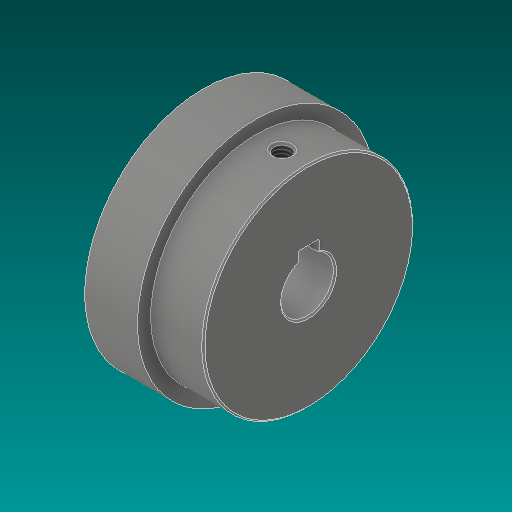
# Autodesk Inventor part: GEYK1.0-70-10-B-10K.0_b
Saved by Autodesk Inventor 2020 (Build 240168000, 168)
## iProperties
Created: 2022-11-14
Part Number: GEYK1.0-70-10-B-10K.0_b
Material: Generic
Catalog Web Link: www.cadenas.de
Description: GEY_body-Plastic Bonded Spur Gears
Vendor: MISUMI
Document SubType Name: Modeling
Designer: psAdmin
Manufacturer: MISUMI
Mass: 26.6277 g
Surface Area: 64.7379 cm^2
Volume: 26.6277 cm^3
Density: 1 g/cm^3
Appearance: PSOLRGB-128-128-128
Category: PARTsolutions
Company: MISUMI
PSOL_IDENT_0: {$CADENAS_DATA/23d-libs/misumi/metric/54_spur_gears/gey_.prj},213 {VTYP=3D},{NB=GEYK1.0-70-10-B-10K.
PSOL_IDENT_1: 0_b},{LINA=GEYK1.0-70-10-B-10K.0},{NN=GEY_body},{DATE=07.06.2021 01:25:59},{GEOMDATE=23.08.2016 05:0
PSOL_IDENT_2: 9:00},{VERSION=},{LINEID=10},{WBVAR=SHS,NT,PS,ALT1,ALT2,BS},{WBNUMERIC=NT,BS}  {NB=GEYK1.0-70-10-B-1
PSOL_IDENT_3: 0K.0_b},{LINA=GEYK1.0-70-10-B-10K.0},{KT=DUMMY},{PN=GEYK1.0-70-10-B-10K.0},{SHS=K},{SHSPN=K},{GEAKBH=
PSOL_IDENT_4: 0},{MAT=MC Nylon},{MATC=S25C},{AC=Set Screw},{MOD=1.0},{NT=70},{NTA=30,32,34,35,36,38,40,42,45,48,50
PSOL_IDENT_5: ,52,56,60,70,75},{B=10},{TS=B},{TSA='B','B'},{PS=10K},{PSA= '10N','10N','10K','10K','11N','11N','12N'
PSOL_IDENT_6: ,'12N','13N','13N','14N','14N','15N','15N','16N','16N','17N','17N','18N','18N','19N','19N','20N','20
PSOL_IDENT_7: N','21N','21N','22N','22N','23N','23N','24N','24N'},{PS1= '10','10','11','11','12','12','13','13','1
PSOL_IDENT_8: 4','14','15','15','16','16','17','17','18','18','19','19','20','20','21','21','22','22','23','23','2
PSOL_IDENT_9: 4','24','25','25','26','26','27','27','28','28'},{PS2= '10N','10N','10K','10K','11N','11N','12N','12
PSOL_IDENT_10: N','13N','13N','14N','14N','15N','15N','16N','16N','17N','17N','18N','18N','19N','19N','20N','20N','
PSOL_IDENT_11: 21N','21N','22N','22N','23N','23N','24N','24N'},{P=10.00},{DD=70.0},{D=72.0},{H=40},{E=45},{L=20},{L
PSOL_IDENT_12: L1=10},{LL2=5.000},{M=M4},{M2=4},{ACSS=M4x3},{TT=1.8},{BB=4},{ALT1=},{ALTA='','w/o Set Screw', '-KC9
PSOL_IDENT_13: 0', 'with KC90 (Set Screw)', '-KC120', 'with KC120 (Set Screw)'},{SCREWL=3},{PLANE=20},{PLANE1=20},{
PSOL_IDENT_14: ALT2=},{ALT2A='','w/o Boss Cut','-BS','with BS (Boss Cut)'},{BS=0.0},{BSA=0},{BSMIN=7.0},{BSMAX=9.5}
PSOL_IDENT_15: ,{HD=15.000}
NB: GEYK1.0-70-10-B-10K.0_b
NN: GEY_body
NT: 70
NBSYN: $PN._b
LINA: GEYK1.0-70-10-B-10K.0
CATALOG: Misumi
PN: GEYK1.0-70-10-B-10K.0
SHS: Key Groove Hole+Tap
MAT: MC Nylon
MATC: S25C
MOD: 1.0
B: 10
PS: 10K
L: 20
LL1: 10
ALT1: w/o Set Screw
ALT2: w/o Boss Cut
BS: 0
SUPPLIER: MISUMI
ARTICLENO: GEYK1.0-70-10-B-10K.0_b
BOMINFO: GEYK1.0-70-10-B-10K.0
CREATOR: CADENAS GmbH
d9: 0.000 mm
Title: GEYK1.0-70-10-B-10K.0
Author: Cadenas PARTsolutions
Comments: Plastic Bonded Spur Gears
Autodesk Inventor part; units mm, degrees
ref_plane "YZ Plane" through (0, 0, 0) normal (1, 0, 0) x (0, 1, 0)
ref_plane "XZ Plane" through (0, 0, 0) normal (0, 1, 0) x (-1, 0, 0)
ref_plane "XY Plane" through (0, 0, 0) normal (0, 0, 1) x (1, 0, 0)
sketch "Sketch_11" plane through (0, 0, 0) normal (0, 0, 1) x (1, 0, 0)
  line L0 (20, 0) -> (0, 0)
  line L1 (0, 0) -> (0, 34)
  line L2 (0, 34) -> (0.5359, 36)
  line L3 (0.5359, 36) -> (9.4641, 36)
  line L4 (9.4641, 36) -> (10, 34)
  line L5 (10, 34) -> (10, 20)
  line L6 (10, 20) -> (19.7, 20)
  line L7 (19.7, 20) -> (20, 19.7)
  line L8 (20, 19.7) -> (20, 0)
  line L9 (20, 0) -> (0, 0)
  constraints: 20 end point
revolve "Revolution1" add sketch "Sketch_11" angle 360 about axis through (20, 0, 0) along (1, 0, 0)
sketch "Sketch_2" plane through (0, 0, 0) normal (1, 0, 0) x (0, 1, 0)
  circle A0 centre (0, 0) radius 41
  circle A1 centre (0, 0) radius 22.5
  constraints: 2 centre point
extrude "Extrusion1" cut sketch "Sketch_2" along normal blind 10
sketch "_____1" plane through (0, 0, 0) normal (0, 0, 1) x (1, 0, 0)
  line L0 (40, 0) -> (-40, 0)
  line L1 (0, 0) -> (0, 5.3)
  line L2 (0, 5.3) -> (0.3, 5)
  line L3 (0.3, 5) -> (19.7, 5)
  line L4 (19.7, 5) -> (20, 5.3)
  line L5 (20, 5.3) -> (20, 0)
  line L6 (20, 0) -> (0, 0)
  constraints: 14 end point
revolve "Revolution2" cut sketch "_____1" angle 360 about axis through (40, 0, 0) along (1, 0, 0)
sketch "Sketch_3" plane through (0, 0, 0) normal (0, 0, 1) x (1, 0, 0)
  line L0 (15, 0) -> (15, 21)
  line L1 (15, 21) -> (17, 21)
  line L2 (17, 21) -> (17, 20)
  line L3 (17, 20) -> (16.621, 19.621)
  line L4 (16.621, 19.621) -> (16.621, 0)
  line L5 (16.621, 0) -> (15, 0)
  line L6 (15, 0) -> (15, 21)
  constraints: 14 end point
revolve "Revolution3" cut sketch "Sketch_3" angle 360 about axis through (15, 0, 0) along (0, -1, 0)
thread "Thread1" size "M4x0.7" class "6H" standard "ISO Metric profile" full length
sketch "Sketch_5" plane through (0, 0, 0) normal (1, 0, 0) x (0, 1, 0)
  line L0 (6.6, 2) -> (0, 2)
  line L1 (0, 2) -> (0, -2)
  line L2 (0, -2) -> (6.6, -2)
  arc A0 (6.6, -2) -> (6.8, -1.8) centre (6.6, -1.8) ccw
  line L3 (6.8, -1.8) -> (6.8, 1.8)
  arc A1 (6.8, 1.8) -> (6.6, 2) centre (6.6, 1.8) ccw
  constraints: 8 end point, 4 point on circle, 2 centre point
extrude "Extrusion2" cut sketch "Sketch_5" along normal blind 20
ref_plane "body_to_teeth_XY" through (0, 0, 0) normal (1, 0, 0) x (0, 0, -1)
ref_plane "body_to_teeth_YZ" through (0, 0, 0) normal (0, 0, -1) x (0, 1, 0)
ref_plane "body_to_teeth_ZX" through (0, 0, 0) normal (0, 1, 0) x (1, 0, 0)
ref_plane "screw1_XY" through (15, 20, 0) normal (0, -1, 0) x (1, 0, 0)
ref_plane "screw1_YZ" through (15, 20, 0) normal (1, 0, 0) x (0, 0, 1)
ref_plane "screw1_ZX" through (15, 20, 0) normal (0, 0, 1) x (0, -1, 0)
ref_plane "screw2_XY" through (15, 0, -20) normal (0, 0, -1) x (1, 0, 0)
ref_plane "screw2_YZ" through (15, 0, -20) normal (1, 0, 0) x (0, -1, 0)
ref_plane "screw2_ZX" through (15, 0, -20) normal (0, -1, 0) x (0, 0, -1)
ref_plane "screw3_XY" through (15, -10, -17.3205) normal (0, -0.5, -0.8660254) x (1, 0, 0)
ref_plane "screw3_YZ" through (15, -10, -17.3205) normal (1, 0, 0) x (0, -0.8660254, 0.5)
ref_plane "screw3_ZX" through (15, -10, -17.3205) normal (0, -0.8660254, 0.5) x (0, -0.5, -0.8660254)
body "Solid1"
